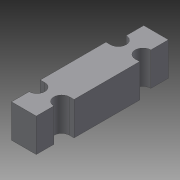
# Autodesk Inventor part: Carriage_Joint_Boltblock_Brace
Saved by Autodesk Inventor 2014 (Build 180170000, 170)
## iProperties
Created: 2014-11-10
Part Number: Carriage_Joint_Boltblock_Brace
Material: Generic
Document SubType Name: Modeling
Designer: ThatOtherGuy
Density: 1 g/cm^3
Appearance: Default
Author: ThatOtherGuy
Autodesk Inventor part; units mm, degrees
ref_plane "YZ Plane" through (0, 0, 0) normal (1, 0, 0) x (0, 1, 0)
ref_plane "XZ Plane" through (0, 0, 0) normal (0, 1, 0) x (-1, 0, 0)
ref_plane "XY Plane" through (0, 0, 0) normal (0, 0, 1) x (1, 0, 0)
sketch "Sketch1" plane through (0, 0, 0) normal (0, 0, 1) x (1, 0, 0)
  line L0 (0, 0) -> (0.9125, 0)
  line L1 (0.9125, 0) -> (0.9125, -6.731)
  line L2 (0.9125, -6.731) -> (5.9125, -6.731)
  line L3 (5.9125, -6.731) -> (5.9125, 0)
  line L4 (5.9125, 0) -> (6.825, 0)
  line L5 (6.825, 0) -> (6.825, 13.269)
  line L6 (6.825, 13.269) -> (5.9125, 13.269)
  line L7 (5.9125, 13.269) -> (5.9125, 20)
  line L8 (5.9125, 20) -> (0.9125, 20)
  line L9 (0.9125, 20) -> (0.9125, 13.269)
  line L10 (0.9125, 13.269) -> (0, 13.269)
  line L11 (0, 13.269) -> (0, 0)
  dimension "d0" = 5
  dimension "d1" = 13.269
  dimension "d2" = 6.731
  dimension "d3" = 6.825
  constraints: 24 end point, 8 parallel, 6 equal length, 2 collinear, 1 horizontal, 1 perpendicular
  measures "d0" distance of L1.end L2.end
  measures "d1" distance of L10.end L0.start
  measures "d2" distance of L2.end L3.end
  measures "d3" distance between parallel lines of L11 L5
extrude "Extrusion1" add sketch "Sketch1" along normal blind 6.731
sketch "Sketch3" plane through (0, 0, 0) normal (0, 0, -1) x (-1, 0, 0)
  line L0 (0, 0) -> (-0.9125, 0) projected
  line L1 (-0.9125, 13.269) -> (0, 13.269) projected
  line L2 (-0.9125, 20) -> (-0.9125, 13.269) projected
  line L3 (-5.9125, 13.269) -> (-5.9125, 20) projected
  line L4 (-6.825, 13.269) -> (-5.9125, 13.269) projected
  line L5 (-5.9125, 0) -> (-6.825, 0) projected
  line L6 (-5.9125, -6.731) -> (-5.9125, 0) projected
  line L7 (-0.9125, 0) -> (-0.9125, -6.731) projected
  arc A0 (-0.9125, 0) -> (-0.9125, -3.176) centre (-0.9125, -1.588) ccw
  arc A1 (-5.9125, -3.176) -> (-5.9125, 0) centre (-5.9125, -1.588) ccw
  arc A2 (-5.9125, 13.269) -> (-5.9125, 16.445) centre (-5.9125, 14.857) ccw
  arc A3 (-0.9125, 16.445) -> (-0.9125, 13.269) centre (-0.9125, 14.857) ccw
  dimension "d13" = 1.588
  constraints: 8 point on circle, 4 centre point, 4 point on line, 4 tangent, 3 equal radius
  measures "d13" radius of A0
extrude "Extrusion3" cut sketch "Sketch3" against normal up to next
equation "\"d2\" = THICKB"
equation "\"d4\" = THICKB"
equation "\"THICKA\" = 3.175"
equation "\"THICKB\" = 6.731"
equation "\"THICKC\" = 12.7"
equation "\"THICKPLY\" = 5"
equation "\"MAGDIA\" = 9.5"
equation "\"BALLDIA\" = 12"
body "Solid1"
